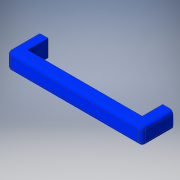
# Autodesk Inventor part: Bumper
Saved by Autodesk Inventor 2016 (Build 200138000, 138)
## iProperties
Created: 2017-01-27
Part Number: Bumper
Material: Generic
Document SubType Name: Modeling
Designer: hamblettk
Density: 1 g/cm^3
Appearance: Default
Author: hamblettk
Autodesk Inventor part; units mm, degrees
ref_plane "YZ Plane" through (0, 0, 0) normal (1, 0, 0) x (0, 1, 0)
ref_plane "XZ Plane" through (0, 0, 0) normal (0, 1, 0) x (-1, 0, 0)
ref_plane "XY Plane" through (0, 0, 0) normal (0, 0, 1) x (1, 0, 0)
sketch "Sketch1" plane through (0, 0, 0) normal (0, 1, 0) x (-1, 0, 0)
  line L0 (0, 0) -> (0, -228.6)
  line L1 (0, -228.6) -> (76.2, -228.6)
  line L2 (76.2, -228.6) -> (76.2, -76.2)
  line L3 (76.2, -76.2) -> (927.1, -76.2)
  line L4 (927.1, -76.2) -> (927.1, -228.6)
  line L5 (927.1, -228.6) -> (1003.3, -228.6)
  line L6 (1003.3, -228.6) -> (1003.3, 0)
  line L7 (1003.3, 0) -> (0, 0)
  dimension "d0" = 228.6
  dimension "d1" = 76.2
  dimension "d2" = 152.4
  dimension "d3" = 850.9
  dimension "d4" = 152.4
  dimension "d5" = 76.2
  constraints: 16 end point, 4 perpendicular, 2 horizontal, 2 vertical
  measures "d0" distance of L0.start L0.end
  measures "d1" distance of L0.end L1.end
  measures "d2" distance of L1.end L2.end
  measures "d3" distance of L2.end L3.end
  measures "d4" distance of L3.end L4.end
  measures "d5" distance of L4.end L5.end
extrude "Extrusion1" add sketch "Sketch1" along normal blind 127
fillet "Fillet1" radius 25.4 8 edges at (-501.65, 127, 0) (-501.65, 0, 0) (0, 127, -114.3) (0, 0, -114.3) (0, 63.5, 0) (-1003.3, 63.5, 0) (-1003.3, 127, -114.3) (-1003.3, 0, -114.3)
body "Solid1"
